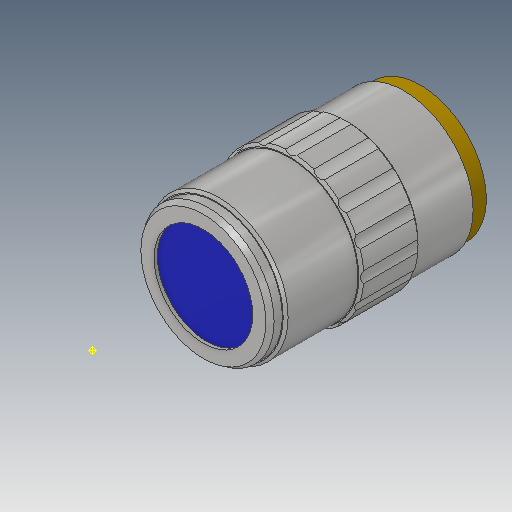
# Autodesk Inventor part: BD-Plan-Apo-approx
Saved by Autodesk Inventor 2021 (Build 250183000, 183)
## iProperties
Created: 2022-09-08
Part Number: BD-Plan-Apo-approx
Material: Generic
Document SubType Name: Modeling
Designer: Nikita
Density: 1 g/cm^3
Appearance: Default
Author: Nikita
Autodesk Inventor part; units mm, degrees
ref_plane "YZ Plane" through (0, 0, 0) normal (1, 0, 0) x (0, 1, 0)
ref_plane "XZ Plane" through (0, 0, 0) normal (0, 1, 0) x (-1, 0, 0)
sketch "Sketch1" plane through (0, 0, 0) normal (0, 0, 1) x (1, 0, 0)
  circle A0 centre (0, 0) radius 19.5
  circle A1 centre (0, 0) radius 20
  circle A2 centre (0, 0) radius 21
  dimension "d0" = 39
  dimension "d1" = 40
  dimension "d2" = 42
  constraints: 3 centre point, 3 coincident
  measures "d0" diameter of A0
  measures "d1" diameter of A1
  measures "d2" diameter of A2
extrude "Extrusion1" add sketch "Sketch1" along normal blind 4 contours A0 | A1
extrude "Extrusion3" add sketch "Sketch1" against normal blind 57 contours A0 | A1 | A2
chamfer "Chamfer2" distance 1 distance2 1.5 1 edges at (-20, 0, 4) measured on face at (-19.5, 0, 4)
chamfer "Chamfer3" distance 0.75 angle 45 1 edges at (-21, 0, 0)
sketch "Sketch2" plane through (0, 0, 4) normal (0, 0, 1) x (1, 0, 0)
  circle A0 centre (0, 0) radius 15
  dimension "d18" = 30
  constraints: 1 centre point, 1 coincident
  measures "d18" diameter of A0
extrude "Extrusion4" cut sketch "Sketch2" against normal blind 1
sketch "Sketch3" plane through (0, 0, -57) normal (0, 0, -1) x (-1, 0, 0)
  circle A0 centre (0, 0) radius 20
  dimension "d21" = 40
  constraints: 1 centre point, 1 coincident
  measures "d21" diameter of A0
extrude "Extrusion5" add sketch "Sketch3" along normal blind 5
ref_plane "Work Plane1" through (0, 0, -22) normal (0, 0, 1) x (1, 0, 0)
sketch "Sketch4" plane through (0, 0, -22) normal (0, 0, 1) x (1, 0, 0)
  circle A0 centre (0, 0) radius 22
  circle A1 centre (0, 0) radius 25
  circle A2 centre (0, 25) radius 3.5
  dimension "d28" = 50
  dimension "d25" = 44
  dimension "d29" = 7
  constraints: 3 coincident, 2 centre point, 1 vertical alignment, 2 other
  measures "d25" diameter of A0
  measures "d29" diameter of A2
extrude "Extrusion6" add sketch "Sketch4" against normal blind 18 contours A0 A2 | A2 A0
extrude "Extrusion7" cut sketch "Sketch4" against normal blind 18 contours A2 A0 | A0 A2 A1 | A1 A2 picked at (-0.1174, 21.8344) picked at (-0.1879, 23.9794)
chamfer "Chamfer4" distance 0.75 angle 45 2 edges at (0, -22, -22) (0, -22, -40)
pattern_circular "Circular Pattern2" count 16 over 360 about axis through (0, 0, -0.75) along (0, 0, 1) of "Extrusion7"
ref_plane "Work Plane2" through (0, 0, 38) normal (0, 0, 1) x (1, 0, 0)
body "Solid1"
